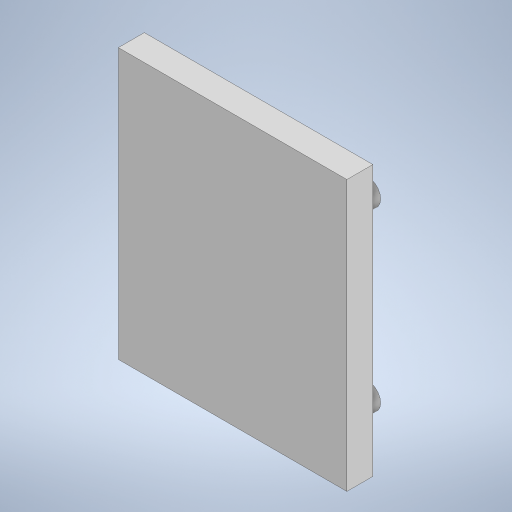
# Autodesk Inventor part: board_setter_cover
Saved by Autodesk Inventor 2024.1 (Build 281209000, 209)
## iProperties
Created: 2024-10-09
Part Number: board_setter_cover
Material: 一般
Document SubType Name: Modeling
Designer: hibik
Density: 1 g/cm^3
Appearance: 既定
Author: hibik
Autodesk Inventor part; units mm, degrees
ref_plane "YZ Plane" through (0, 0, 0) normal (1, 0, 0) x (0, 1, 0)
ref_plane "XZ Plane" through (0, 0, 0) normal (0, 1, 0) x (-1, 0, 0)
ref_plane "XY Plane" through (0, 0, 0) normal (0, 0, 1) x (1, 0, 0)
sketch "スケッチ1" plane through (0, 0, 0) normal (0, 0, 1) x (1, 0, 0)
  line L0 (22, 24) -> (-22, 24)
  line L1 (-22, 24) -> (-22, -24)
  line L2 (-22, -24) -> (22, -24)
  line L3 (22, -24) -> (22, 24)
  line L4 (22, 24) -> (-22, -24) construction
  line L5 (-22, 24) -> (22, -24) construction
  line L6 (-17, 15) -> (17, 15) construction
  line L7 (17, 15) -> (17, -19) construction
  line L8 (17, -19) -> (-17, -19) construction
  line L9 (-17, -19) -> (-17, 15) construction
  circle A0 centre (-17, 15) radius 2.5
  circle A1 centre (17, 15) radius 2.5
  circle A2 centre (17, -19) radius 2.5
  circle A3 centre (-17, -19) radius 2.5
  line L10 (22, -24) -> (-22, -24)
  line L11 (-22, -24) -> (-22, -28)
  line L12 (-22, -28) -> (22, -28)
  line L13 (22, -28) -> (22, -24)
  point P0 (0, 0)
  point P1 (0, 15)
  point P2 (0, 24)
  dimension "d0" = 48
  dimension "d1" = 44
  dimension "d2" = 34
  dimension "d3" = 5
  dimension "d4" = 5
  dimension "d5" = 5
  dimension "d16" = 4
  constraints: 28 end point, 6 parallel, 4 centre point, 4 coincident, 4 midpoint, 4 perpendicular, 3 equal radius, 3 horizontal, 1 collinear, 1 vertical alignment
  measures "d0" distance of L0.end L1.end
  measures "d1" distance of L0.start L0.end
  measures "d2" distance of L7.end L8.end
  measures "d3" distance between parallel lines of L1 L9
  measures "d4" distance between parallel lines of L2 L8
  measures "d5" diameter of A0
  measures "d16" distance of L11.end L10.end
extrude "押し出し1" add sketch "スケッチ1" along normal blind 5 contours L3 L2 L1 L0 | L13 L12 L11 L2 | A0 | A1 | A2 | A3
extrude "押し出し2" add sketch "スケッチ1" against normal blind 4 contours A0 | A1 | A2 | A3
equation "\"d4\" = d3"
